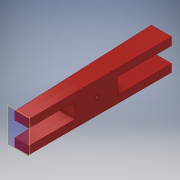
# Autodesk Inventor part: jigForRipCutsB
Saved by Autodesk Inventor 2019.1 (Build 231200000, 200)
## iProperties
Created: 2018-07-31
Part Number: jigForRipCutsB
Material: PC/ABS Plastic
Document SubType Name: Modeling
Designer: steele
Density: 0.357273 g/cm^3
Appearance: Orange-Red
Author: steele
Autodesk Inventor part; units mm, degrees
ref_plane "YZ Plane" through (0, 0, 0) normal (1, 0, 0) x (0, 1, 0)
ref_plane "XZ Plane" through (0, 0, 0) normal (0, 1, 0) x (-1, 0, 0)
sketch "Sketch1" plane through (0, 0, 0) normal (0, 1, 0) x (-1, 0, 0)
  line L0 (0, 0) -> (0, -469.9)
  line L1 (0, -469.9) -> (0, -122.0086)
  line L2 (0, -469.9) -> (20.5163, -469.9)
  line L3 (20.5163, -469.9) -> (0, 0)
  dimension "d0" = 469.9
  dimension "d1" = 2.5
  constraints: 8 end point, 1 horizontal, 1 point on line, 1 vertical
  measures "d0" distance of L0.start L0.end
  measures "d1" angle of L3 L0
extrude "Extrusion1" add sketch "Sketch1" along normal blind 50.8
ref_plane "Work Plane1" through (-20.5163, 50.8, -469.9) normal (1, 0, 0) x (0, 0, -1)
sketch "Sketch2" plane through (0, 0, 0) normal (1, 0, 0) x (0, 0, -1)
  line L0 (0, 0) -> (469.9, 0) projected
  line L1 (0, 50.8) -> (469.9, 50.8) projected
  line L2 (0, 0) -> (469.9, 0)
  line L3 (469.9, 0) -> (469.9, 50.8)
  line L4 (469.9, 50.8) -> (0, 50.8)
  line L5 (0, 50.8) -> (0, 0)
  constraints: 8 end point, 2 parallel, 1 horizontal, 1 perpendicular
extrude "Extrusion2" add sketch "Sketch2" along normal blind 12.7
sketch "Sketch4" plane through (-20.5163, 50.8, -469.9) normal (1, 0, 0) x (0, 0, -1)
  line L0 (0, -50.8) -> (0, 0) construction
  line L1 (0, -25.4) -> (-279.4, -25.4) construction
  line L2 (0, -50.8) -> (-469.9, -50.8) construction
  line L3 (-469.9, -50.8) -> (-469.9, 0) construction
  point P0 (-381, -25.4)
  point P1 (-123.825, -25.4)
  point P2 (-469.9, 0)
  dimension "d16" = 25.4
  dimension "d17" = 88.9
  dimension "d18" = 346.075
  constraints: 2 end point, 2 point on line, 1 horizontal, 1 midpoint, 1 other
  measures "d16" distance between parallel lines of L1 L2
hole "Hole2" at (-20.5163, 25.4, -88.9) at (-20.5163, 25.4, -346.075) direction (1, 0, 0) diameter 6.7564 end through all clearance for "Flat Head Machine Screw (82)" size "1/4" standard "Ansi Unified Screw Threads"
sketch "Sketch6" plane through (-20.5163, 50.8, -469.9) normal (1, 0, 0) x (0, 0, -1)
  circle A0 centre (-123.825, -25.4) radius 3.3782 projected
  line L0 (-130.2408, -25.4) -> (-127.0329, -19.8438)
  line L1 (-127.0329, -19.8438) -> (-120.6171, -19.8438)
  line L2 (-120.6171, -19.8438) -> (-117.4092, -25.4)
  line L3 (-117.4092, -25.4) -> (-120.6171, -30.9563)
  line L4 (-120.6171, -30.9563) -> (-127.0329, -30.9562)
  line L5 (-127.0329, -30.9562) -> (-130.2408, -25.4)
  circle A1 centre (-381, -25.4) radius 3.3782 projected
  line L6 (-387.4158, -25.4) -> (-384.2079, -19.8438)
  line L7 (-384.2079, -19.8438) -> (-377.7921, -19.8438)
  line L8 (-377.7921, -19.8438) -> (-374.5842, -25.4)
  line L9 (-374.5842, -25.4) -> (-377.7921, -30.9563)
  line L10 (-377.7921, -30.9563) -> (-384.2079, -30.9563)
  line L11 (-384.2079, -30.9563) -> (-387.4158, -25.4)
  line L12 (0, 0) -> (-469.9, 0) projected
  point P0 (-469.9, -50.8)
  dimension "d26" = 11.1125
  constraints: 24 end point, 2 coincident, 1 collinear, 1 parallel, 26 other
  measures "d26" distance between parallel lines of L4 L1
extrude "Extrusion3" cut sketch "Sketch6" along normal blind 23.368
ref_plane "Work Plane2" through (-20.5163, 0, -234.95) normal (0, 0, -1) x (-1, 0, 0)
split "Split2" plane through (-20.5163, 0, -234.95) removes the side toward (0, 0, 1)
sketch "Sketch7" plane through (-20.5163, 50.8, -469.9) normal (1, 0, 0) x (0, 0, -1)
  line L0 (-158.75, -38.1) -> (-311.15, -38.1)
  line L1 (-311.15, -38.1) -> (-311.15, -12.7)
  line L2 (-311.15, -12.7) -> (-158.75, -12.7)
  line L3 (-158.75, -12.7) -> (-158.75, -38.1)
  line L4 (-234.95, 0) -> (-234.95, -50.8) projected
  line L5 (-158.75, -38.1) -> (-311.15, -12.7) construction
  line L6 (-311.15, -38.1) -> (-158.75, -12.7) construction
  line L7 (88.9, -38.1) -> (-88.9, -38.1)
  line L8 (-88.9, -38.1) -> (-88.9, -12.7)
  line L9 (-88.9, -12.7) -> (88.9, -12.7)
  line L10 (88.9, -12.7) -> (88.9, -38.1)
  line L11 (0, -50.8) -> (0, 0) projected
  line L12 (88.9, -38.1) -> (-88.9, -12.7) construction
  line L13 (-88.9, -38.1) -> (88.9, -12.7) construction
  point P0 (-469.9, -50.8)
  point P1 (-234.95, -25.4)
  point P2 (0, -25.4)
  dimension "d30" = 25.4
  dimension "d31" = 177.8
  dimension "d32" = 152.4
  constraints: 24 end point, 6 midpoint, 5 parallel, 4 perpendicular
  measures "d30" distance of L7.end L8.end
  measures "d31" distance of L8.end L9.end
  measures "d32" distance of L1.end L2.end
extrude "Extrusion4" cut sketch "Sketch7" along normal through all
equation "\"d0\" = lengthOfFixture"
equation "\"d1\" = cutAngle"
equation "\"d2\" = heightOfJig"
equation "\"d4\" = addedDepthToSupportBolts"
equation "\"d16\" = heightOfBoltHolt"
equation "\"d17\" = bottomToFirstHole"
equation "\"d18\" = bottomToSecondHole"
equation "\"d26\" = hexBoltDiameter"
equation "\"d27\" = depthOfHoleForHexBolt + clearanceForHexbolt"
equation "\"lengthOfFixture\" = 469.9"
equation "\"cutAngle\" = 2.5deg"
equation "\"bottomToFirstHole\" = 88.9"
equation "\"distanceBetweenBolts\" = 257.175"
equation "\"bottomToSecondHole\" = bottomToFirstHole + distanceBetweenBolts"
equation "\"heightOfBoltHolt\" = 25.4"
equation "\"boltSize\" = 6.35"
equation "\"heightOfJig\" = 50.8"
equation "\"addedDepthToSupportBolts\" = 12.7"
equation "\"depthOfHoleForHexBolt\" = 22.86"
equation "\"hexBoltDiameter\" = 11.1125"
equation "\"clearanceForHexbolt\" = 0.508"
equation "\"d29\" = -0.5 * lengthOfFixture"
body "Solid1"
